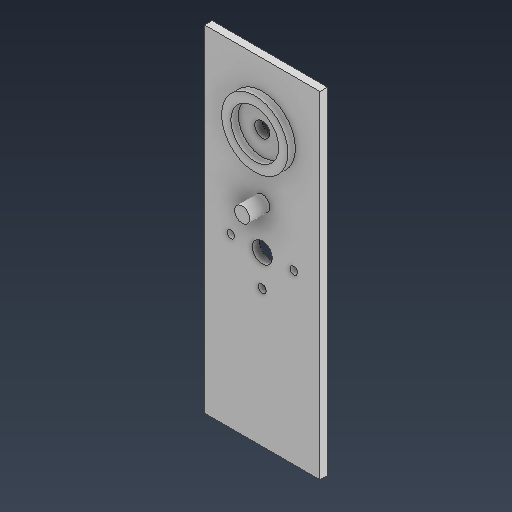
# Autodesk Inventor part: пластина для редуктора
Saved by Autodesk Inventor 2025 (Build 290162000, 162)
## iProperties
Created: 2025-09-21
Part Number: пластина для редуктора
Material: Типовые
Document SubType Name: Modeling
Designer: GameHD
Density: 1 g/cm^3
Appearance: По умолчанию
Author: GameHD
Autodesk Inventor part; units mm, degrees
ref_plane "YZ Plane" through (0, 0, 0) normal (1, 0, 0) x (0, 1, 0)
ref_plane "XZ Plane" through (0, 0, 0) normal (0, 1, 0) x (-1, 0, 0)
ref_plane "XY Plane" through (0, 0, 0) normal (0, 0, 1) x (1, 0, 0)
sketch "Эскиз1" plane through (0, 0, 0) normal (0, 0, 1) x (1, 0, 0)
  circle A0 centre (0.9164, -10.9801) radius 1.6008
  arc A1 (-10.5243, 2.5819) -> (-10.0836, 1.5104) centre (-11.5836, 1.5199) ccw
  arc A2 (12.3571, 0.4579) -> (11.9164, 1.5294) centre (13.4164, 1.5199) ccw
  circle A3 centre (-11.5836, 1.5199) radius 1.5
  circle A4 centre (13.4164, 1.5199) radius 1.5
  line L0 (-21.9797, -65.2227) -> (23.8125, -65.2227)
  line L1 (23.8125, -65.2227) -> (23.8125, 68.2625)
  line L2 (23.8125, 68.2625) -> (-21.9797, 68.2625)
  line L3 (-21.9797, 68.2625) -> (-21.9797, -65.2227)
  line L4 (-21.9797, -65.2227) -> (23.8125, 68.2625) construction
  line L5 (23.8125, -65.2227) -> (-21.9797, 68.2625) construction
  point P0 (0, 0)
  point P1 (-10.0836, 1.5104)
  point P2 (12.3571, 0.4579)
  point P3 (11.9164, 1.5294)
  constraints: 12 end point, 4 centre point, 4 point on circle, 2 coincident, 2 parallel, 1 concentric, 1 horizontal, 1 perpendicular, 4 other
extrude "Выдавливание1" add sketch "Эскиз1" along normal blind 3
sketch "Эскиз2" plane through (0, 0, 3) normal (0, 0, 1) x (1, 0, 0)
  line L0 (23.8125, -65.2227) -> (23.8125, 68.2625) projected
  line L1 (23.8125, 68.2625) -> (-21.9797, 68.2625) projected
  line L2 (-21.9797, 68.2625) -> (-21.9797, -65.2227) projected
  line L3 (-21.9797, -65.2227) -> (23.8125, -65.2227) projected
  circle A0 centre (-11.5836, 1.5199) radius 1.5 projected
  circle A1 centre (13.4164, 1.5199) radius 1.5 projected
  circle A2 centre (0.9164, -10.9801) radius 1.6008 projected
  line L4 (-11.5836, 1.5199) -> (13.4164, 1.5199)
  line L5 (0.9164, 14.0199) -> (0.9164, -10.9801)
  circle A3 centre (0.9164, 1.5199) radius 4
  point P0 (0, 0)
  dimension "d2" = 8
  constraints: 4 end point, 1 centre point, 1 horizontal, 1 midpoint, 1 vertical
  measures "d2" diameter of A3
extrude "Выдавливание2" cut sketch "Эскиз2" against normal blind 3 contours A3 L5 L4 | L4 L5 A3 | L5 A3 L4 | L4 A3 L5
sketch "Эскиз3" plane through (0, 0, 3) normal (0, 0, 1) x (1, 0, 0)
  circle A0 centre (0.9164, 1.5199) radius 4 projected
  line L0 (23.8125, -65.2227) -> (23.8125, 68.2625) projected
  line L1 (23.8125, 68.2625) -> (-21.9797, 68.2625) projected
  line L2 (-21.9797, 68.2625) -> (-21.9797, -65.2227) projected
  line L3 (-21.9797, -65.2227) -> (23.8125, -65.2227) projected
  circle A1 centre (-11.5836, 1.5199) radius 1.5 projected
  circle A2 centre (13.4164, 1.5199) radius 1.5 projected
  circle A3 centre (0.9164, -10.9801) radius 1.6008 projected
  line L4 (0.9164, 1.5199) -> (0.9164, 18.5199)
  circle A4 centre (0.9164, 18.5199) radius 3
  point P0 (0, 0)
  dimension "d5" = 17
  dimension "d6" = 6
  constraints: 2 end point, 1 centre point, 1 coincident, 1 vertical
  measures "d5" distance of L4.start L4.end
  measures "d6" diameter of A4
extrude "Выдавливание3" add sketch "Эскиз3" along normal blind 8 contours A4
sketch "Эскиз4" plane through (0, 0, 3) normal (0, 0, 1) x (1, 0, 0)
  circle A0 centre (0.9164, 18.5199) radius 3 projected
  circle A1 centre (0.9164, 43.7699) radius 9.5
  circle A2 centre (0.9164, 43.7699) radius 13.15
  circle A3 centre (0.9164, 18.5199) radius 3 projected
  circle A4 centre (0.9164, 1.5199) radius 4 projected
  line L0 (23.8125, -65.2227) -> (23.8125, 68.2625) projected
  line L1 (23.8125, 68.2625) -> (-21.9797, 68.2625) projected
  line L2 (-21.9797, 68.2625) -> (-21.9797, -65.2227) projected
  line L3 (-21.9797, -65.2227) -> (23.8125, -65.2227) projected
  circle A5 centre (-11.5836, 1.5199) radius 1.5 projected
  circle A6 centre (13.4164, 1.5199) radius 1.5 projected
  circle A7 centre (0.9164, -10.9801) radius 1.6008 projected
  point P0 (0, 0)
  dimension "d17" = 42.25
  dimension "d18" = 0
  constraints: 2 centre point
  measures "d17" distance of A4.centre A1.centre
  measures "d18" distance of A1.centre A2.centre
extrude "Выдавливание4" add sketch "Эскиз4" along normal blind 3 contours A2
sketch "Эскиз5" plane through (0, 0, 3) normal (0, 0, 1) x (1, 0, 0)
  circle A0 centre (0.9164, -10.9801) radius 1.6008 projected
  circle A1 centre (13.4164, 1.5199) radius 1.5 projected
  circle A2 centre (-11.5836, 1.5199) radius 1.5 projected
  line L0 (23.8125, -65.2227) -> (23.8125, 68.2625) projected
  line L1 (23.8125, 68.2625) -> (-21.9797, 68.2625) projected
  line L2 (-21.9797, 68.2625) -> (-21.9797, -65.2227) projected
  line L3 (-21.9797, -65.2227) -> (23.8125, -65.2227) projected
  circle A3 centre (0.9164, 43.7699) radius 13.15 projected
  circle A4 centre (0.9164, 1.5199) radius 4 projected
  circle A5 centre (0.9164, 43.7699) radius 3
  point P0 (0, 0)
  dimension "d12" = 6
  dimension "d16" = 0
  constraints: 1 centre point
  measures "d12" diameter of A5
  measures "d16" distance of A5.centre A3.centre
extrude "Выдавливание5" cut sketch "Эскиз5" against normal blind 8 contours A5
